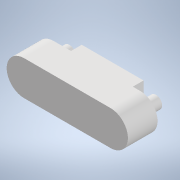
# Autodesk Inventor part: SpringHolderV1
Saved by Autodesk Inventor 2020 (Build 240168000, 168)
## iProperties
Created: 2020-06-07
Part Number: SpringHolderV1
Material: Generic
Document SubType Name: Modeling
Designer: Kitte_x
Density: 1 g/cm^3
Appearance: Default
Author: Kitte_x
Autodesk Inventor part; units mm, degrees
ref_plane "YZ Plane" through (0, 0, 0) normal (1, 0, 0) x (0, 1, 0)
ref_plane "XZ Plane" through (0, 0, 0) normal (0, 1, 0) x (-1, 0, 0)
ref_plane "XY Plane" through (0, 0, 0) normal (0, 0, 1) x (1, 0, 0)
sketch "Sketch1" plane through (0, 0, 0) normal (0, 0, 1) x (1, 0, 0)
  circle A0 centre (17.5, 0) radius 2.5 projected
  circle A1 centre (-17.5, 0) radius 2.5 projected
  line L0 (17.5, -7) -> (-17.5, -7)
  arc A2 (-17.5, 7) -> (-17.5, -7) centre (-17.5, 0) ccw
  line L1 (-17.5, 7) -> (17.5, 7)
  arc A3 (17.5, -7) -> (17.5, 7) centre (17.5, 0) ccw
  line L2 (-12.5, -5) -> (12.5, -5) projected
  line L3 (12.5, 5) -> (-12.5, 5) projected
  circle A4 centre (0, 0) radius 3.5
  dimension "d0" = 2
  dimension "d1" = 17.5
  dimension "d2" = 7
  constraints: 4 end point, 4 point on circle, 4 tangent, 3 centre point, 1 coincident, 1 concentric, 1 horizontal, 1 parallel
  measures "d0" distance between parallel lines of L0 L2
  measures "d1" horizontal distance of point (0, 0) L1.end
  measures "d2" diameter of A4
extrude "Extrusion1" add sketch "Sketch1" along normal blind 10 contours A0 | A1 | L0 A2 L1 A3
sketch "Sketch2" plane through (0, 0, 10) normal (0, 0, 1) x (1, 0, 0)
  arc A0 (17.5, -7) -> (17.5, 7) centre (17.5, 0) ccw projected
  line L0 (-17.5, -7) -> (17.5, -7) projected
  arc A1 (-17.5, 7) -> (-17.5, -7) centre (-17.5, 0) ccw projected
  line L1 (17.5, 7) -> (-17.5, 7) projected
  point P0 (0, 0)
extrude "Extrusion2" add sketch "Sketch2" along normal blind 2
sketch "Sketch3" plane through (0, 0, 10) normal (0, 0, -1) x (-1, 0, 0)
  circle A0 centre (0, 0) radius 1.7
  dimension "d7" = 3.4
  constraints: 1 centre point, 1 coincident
  measures "d7" diameter of A0
extrude "Extrusion3" add sketch "Sketch3" along normal blind 5
sketch "Sketch4" plane through (0, 0, 0) normal (0, 0, -1) x (-1, 0, 0)
  circle A0 centre (17.5, 0) radius 2.5 projected
  line L0 (12.5, 5) -> (12.5, -5) projected
  line L1 (-12.5, 5) -> (12.5, 5) projected
  line L2 (12.5, -5) -> (-12.5, -5) projected
  line L3 (-12.5, -5) -> (-12.5, 5) projected
  circle A1 centre (0, 0) radius 3.5 projected
  circle A2 centre (-17.5, 0) radius 2.5 projected
extrude "Extrusion4" add sketch "Sketch4" along normal blind 6.35
body "Solid1"
